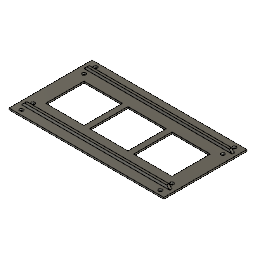
smmb_front-led-matrix (Autodesk Fusion 360 design; units mm, degrees)
Autodesk Fusion 360 part; units mm, degrees
sketch "Sketch3" plane through (0, 0, 0) normal (0, 0, 1) x (1, 0, 0)
  line L0 (0, 0) -> (32, 0)
  line L1 (32, 0) -> (32, 32)
  line L2 (32, 32) -> (0, 32)
  line L3 (0, 32) -> (0, 0)
  line L4 (-0.5, 32.5) -> (-0.5, -0.5)
  line L5 (-0.5, -0.5) -> (32.5, -0.5)
  line L6 (32.5, -0.5) -> (32.5, 32.5)
  line L7 (32.5, 32.5) -> (-0.5, 32.5)
  line L8 (70, 32) -> (38, 32)
  line L9 (38, 32) -> (38, 0)
  line L10 (37.5, -0.5) -> (70.5, -0.5)
  line L11 (70.5, 32.5) -> (37.5, 32.5)
  line L12 (70, 0) -> (70, 32)
  line L13 (70.5, -0.5) -> (70.5, 32.5)
  line L14 (38, 0) -> (70, 0)
  line L15 (37.5, 32.5) -> (37.5, -0.5)
  line L16 (108, 32) -> (76, 32)
  line L17 (76, 32) -> (76, 0)
  line L18 (75.5, -0.5) -> (108.5, -0.5)
  line L19 (108.5, 32.5) -> (75.5, 32.5)
  line L20 (108, 0) -> (108, 32)
  line L21 (108.5, -0.5) -> (108.5, 32.5)
  line L22 (76, 0) -> (108, 0)
  line L23 (75.5, 32.5) -> (75.5, -0.5)
  line L24 (38, 32) -> (70, 0)
  line L25 (70, 32) -> (38, 0)
  line L26 (118, -10) -> (-10, -10)
  line L27 (-10, -10) -> (-10, 42)
  line L28 (-10, 42) -> (118, 42)
  line L29 (118, 42) -> (118, -10)
  line L30 (118, -10) -> (-10, 42) construction
  line L31 (-10, -10) -> (118, 42) construction
  circle A0 centre (3, 26) radius 2.05
  circle A1 centre (3, 26) radius 3.55
  circle A2 centre (29, 26) radius 3.55
  circle A3 centre (29, 26) radius 2.05
  circle A4 centre (29, 6) radius 2.05
  circle A5 centre (29, 6) radius 3.55
  circle A6 centre (3, 6) radius 2.05
  circle A7 centre (3, 6) radius 3.55
  circle A8 centre (67, 6) radius 2.05
  circle A9 centre (67, 6) radius 3.55
  circle A10 centre (41, 6) radius 2.05
  circle A11 centre (41, 6) radius 3.55
  circle A12 centre (67, 26) radius 2.05
  circle A13 centre (67, 26) radius 3.55
  circle A14 centre (41, 26) radius 2.05
  circle A15 centre (41, 26) radius 3.55
  circle A16 centre (105, 6) radius 2.05
  circle A17 centre (105, 6) radius 3.55
  circle A18 centre (79, 6) radius 2.05
  circle A19 centre (79, 6) radius 3.55
  circle A20 centre (105, 26) radius 2.05
  circle A21 centre (105, 26) radius 3.55
  circle A22 centre (79, 26) radius 2.05
  circle A23 centre (79, 26) radius 3.55
  line L32 (3, 22.45) -> (-0.5, 22.45)
  line L33 (-0.5, 22.45) -> (-0.5, 9.55)
  line L34 (-0.5, 9.55) -> (3, 9.55)
  line L35 (3, 9.55) -> (3, 22.45)
  line L36 (41, 22.45) -> (37.5, 22.45)
  line L37 (41, 9.55) -> (41, 22.45)
  line L38 (37.5, 9.55) -> (41, 9.55)
  line L39 (37.5, 22.45) -> (37.5, 9.55)
  line L40 (79, 22.45) -> (75.5, 22.45)
  line L41 (79, 9.55) -> (79, 22.45)
  line L42 (75.5, 9.55) -> (79, 9.55)
  line L43 (75.5, 22.45) -> (75.5, 9.55)
  circle A24 centre (-6, 38) radius 1.55
  circle A25 centre (-6, 38) radius 3.05
  circle A26 centre (54, 38) radius 1.55
  circle A27 centre (54, 38) radius 3.05
  circle A28 centre (114, 38) radius 1.55
  circle A29 centre (114, 38) radius 3.05
  circle A30 centre (-6, -6) radius 1.55
  circle A31 centre (-6, -6) radius 3.05
  circle A32 centre (54, -6) radius 1.55
  circle A33 centre (54, -6) radius 3.05
  circle A34 centre (114, -6) radius 1.55
  circle A35 centre (114, -6) radius 3.05
  line L44 (121, -20) -> (-13, -20)
  line L45 (-13, -20) -> (-13, 52)
  line L46 (-13, 52) -> (121, 52)
  line L47 (121, 52) -> (121, -20)
  line L48 (121, -20) -> (-13, 52) construction
  line L49 (-13, -20) -> (121, 52) construction
  circle A36 centre (-6, 48) radius 1.55
  circle A37 centre (114, 48) radius 1.55
  circle A38 centre (114, -16) radius 1.55
  circle A39 centre (-6, -16) radius 1.55
  line L50 (118, 15) -> (-10, 15)
  line L51 (-10, 15) -> (-10, 17)
  line L52 (-10, 17) -> (118, 17)
  line L53 (118, 17) -> (118, 15)
  line L54 (118, 15) -> (-10, 17) construction
  line L55 (-10, 15) -> (118, 17) construction
  line L56 (-10, -10) -> (118, -10)
  line L57 (118, -10) -> (118, -12)
  line L58 (118, -12) -> (-10, -12)
  line L59 (-10, -12) -> (-10, -10)
  line L60 (-10, 42) -> (118, 42)
  line L61 (118, 42) -> (118, 44)
  line L62 (118, 44) -> (-10, 44)
  line L63 (-10, 44) -> (-10, 42)
  point P0 (38, 0)
  point P1 (76, 0)
  point P2 (54, 16)
  point P3 (54, 16)
  point P4 (54, 16)
  dimension "d57" = 32
  dimension "d58" = 32
  dimension "d59" = 0.5
  dimension "d62" = 76
  dimension "d63" = 0
  dimension "d66" = 10
  dimension "d67" = 10
  dimension "d68" = 4.1
  dimension "d69" = 3
  dimension "d70" = 6
  dimension "d71" = 7.1
  dimension "d74" = 26
  dimension "d75" = 0
  dimension "d78" = 0
  dimension "d79" = -20
  dimension "d82" = 76
  dimension "d83" = 0
  dimension "d84" = 3.5
  dimension "d85" = 12.9
  dimension "d86" = 9.55
  dimension "d89" = 76
  dimension "d90" = 0
  dimension "d95" = 4
  dimension "d96" = 4
  dimension "d97" = 3.1
  dimension "d98" = 6.1
  dimension "d101" = 120
  dimension "d102" = 0
  dimension "d105" = 0
  dimension "d106" = -44
  dimension "d114" = 134
  dimension "d115" = 72
  dimension "d116" = 3.1
  dimension "d117" = 7
  dimension "d118" = 4
  dimension "d121" = 120
  dimension "d122" = 0
  dimension "d125" = 0
  dimension "d126" = -64
  dimension "d127" = 128
  dimension "d128" = 2
  dimension "d134" = 2
  dimension "d135" = 2
  constraint horizontal L0
  constraint vertical L1
  constraint horizontal L2
  constraint vertical L3
  constraint coincident L0.start L3.end
  constraint coincident P0 L9.end
  constraint perpendicular L26 L27
  constraint parallel L26 L28
  constraint parallel L27 L29
  constraint horizontal L26
  constraint coincident L30 P4
  constraint coincident L31 P4
  constraint midpoint L24 P4
  constraint concentric A0 A1
  constraint horizontal L32
  constraint vertical L33
  constraint horizontal L34
  constraint vertical L35
  constraint coincident A1 L32.start
  constraint concentric A24 A25
  constraint perpendicular L44 L45
  constraint parallel L44 L46
  constraint parallel L45 L47
  constraint horizontal L44
  constraint coincident L48 P4
  constraint coincident L49 P4
  constraint coincident P4 P3
  constraint perpendicular L50 L51
  constraint parallel L50 L52
  constraint parallel L51 L53
  constraint horizontal L50
  constraint coincident L54 P4
  constraint coincident L55 P4
  measures "d57" distance of L0.start L2.end
  measures "d58" distance of L0.start L0.end
  measures "d66" distance of L2 L28
  measures "d67" distance of L3 L27
  measures "d68" diameter of A0
  measures "d69" distance of L3 A0.centre
  measures "d70" distance of L2 A0.centre
  measures "d71" diameter of A1
  measures "d84" distance of L32.start L32.end
  measures "d85" distance of L32.start L34.end
  measures "d86" distance of L2 L32
  measures "d95" distance of L27 A24.centre
  measures "d96" distance of L28 A24.centre
  measures "d97" diameter of A24
  measures "d98" diameter of A25
  measures "d114" distance of L44.start L44.end
  measures "d115" distance of L44 L46
  measures "d116" diameter of A36
  measures "d117" distance of L45 A36.centre
  measures "d118" distance of L46 A36.centre
  measures "d127" distance of L51.end L52.end
  measures "d128" distance of L50.end L51.end
  measures "d134" distance of L26.end L58.end
  measures "d135" distance of L27.end L62.end
extrude "Extrude4" add sketch "Sketch3" along normal blind 1.5 contours L4 A7 | L4 L5 L6 L10 L13 L15 L18 L21 L23 L26 L27 L29 A5 A7 A9 A11 A17 A19 L33 L39 L43 L50 L56 | L6 A5 | L6 L15 L39 L50 L52 | L4 L27 L33 L50 L51 L52 | L4 L6 L7 L11 L13 L15 L19 L21 L23 L27 L28 L29 A1 A2 A13 A15 A21 A23 L33 L39 L43 L52 L60 | L6 A2 | L26 L56 L57 L58 L59 | L15 A11 | L4 A1 | L28 L60 L61 L62 L63 | L15 A15 | L21 L29 L50 L52 L53 | L21 A17 | L13 A9 | L13 L23 L43 L50 L52 | L21 A21 | L13 A13 | L23 A19 | L23 A23 | A25 | A26 | A27 | A29 | A31 | A32 | A33 | A35 | L44 L45 L46 L47
extrude "Extrude6" add sketch "Sketch3" along normal blind 4 contours L26 L56 L57 L58 L59 | L28 L60 L61 L62 L63
chamfer "Chamfer2" distance 2.5 angle 45 4 edges at (118, 43, 4) (118, -11, 4) (-10, -11, 4) (-10, 43, 4)
extrude "Extrude5" [suppressed]
chamfer "Chamfer1" [suppressed]
equation "d71 = d68 + 3 mm"
equation "d98 = d97 + 3 mm"
equation "d115 = 52 mm + 20 mm"
equation "d116 = d97"
